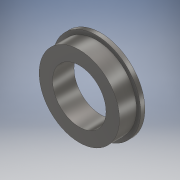
# Autodesk Inventor part: bear_f10_15_sa
Saved by Autodesk Inventor 2018 (Build 220112000, 112)
## iProperties
Created: 2018-03-05
Part Number: bear_f10_15_sa
Material: ステンレス鋼
Document SubType Name: Modeling
Designer: shun
Density: 8 g/cm^3
Appearance: 半つや出し
Author: shun
Autodesk Inventor part; units mm, degrees
ref_plane "YZ Plane" through (0, 0, 0) normal (1, 0, 0) x (0, 1, 0)
ref_plane "XZ Plane" through (0, 0, 0) normal (0, 1, 0) x (-1, 0, 0)
ref_plane "XY Plane" through (0, 0, 0) normal (0, 0, 1) x (1, 0, 0)
sketch "スケッチ1" plane through (0, 0, 0) normal (0, 0, 1) x (1, 0, 0)
  line L0 (5, 0) -> (8.25, 0)
  line L1 (5, 0) -> (5, -4)
  line L2 (5, -4) -> (7.5, -4)
  line L3 (8.25, 0) -> (8.25, -0.8)
  line L4 (7.5, -4) -> (7.5, -0.8)
  line L5 (7.5, -0.8) -> (8.25, -0.8)
  line L6 (0, -4.8) -> (0, 0.8) projected
  point P0 (0, 0)
  dimension "d0" = 5
  dimension "d1" = 3.25
  dimension "d2" = 4
  dimension "d3" = 2.5
  dimension "d4" = 0.8
  constraints: 12 end point, 3 vertical, 2 perpendicular, 1 horizontal
  measures "d0" distance of point (0, 0) L0.start
  measures "d1" distance of L0.start L0.end
  measures "d2" distance of L0.start L1.end
  measures "d3" distance of L1.end L2.end
  measures "d4" distance of L0.end L3.end
revolve "回転1" add sketch "スケッチ1" angle 360 about axis through (0, -10, 0) along (0, 1, 0)
